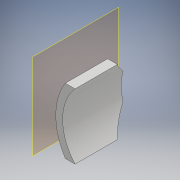
# Autodesk Inventor part: 15mm_radius_mold_with_crystal_skull
Saved by Autodesk Inventor 2018 (Build 220112000, 112)
## iProperties
Created: 2018-06-11
Part Number: 15mm_radius_mold_with_crystal_skull
Material: Generic
Document SubType Name: Modeling
Designer: McCormick Lab
Density: 1 g/cm^3
Appearance: Default
Author: McCormick Lab
Autodesk Inventor part; units mm, degrees
ref_plane "YZ Plane" through (0, 0, 0) normal (1, 0, 0) x (0, 1, 0)
ref_plane "XZ Plane" through (0, 0, 0) normal (0, 1, 0) x (-1, 0, 0)
ref_plane "XY Plane" through (0, 0, 0) normal (0, 0, 1) x (1, 0, 0)
sketch "Sketch1" plane through (0, 0, 0) normal (0, 1, 0) x (-1, 0, 0)
  arc A0 (0, -7.5) -> (0, 7.5) centre (0, 0) ccw
  line L0 (0, 7.5) -> (0, -7.5)
  dimension "d0" = 15
  constraints: 2 end point, 2 point on circle, 1 centre point, 1 coincident, 1 vertical
  measures "d0" diameter of A0
extrude "Extrusion1" add sketch "Sketch1" along normal blind 12
ref_plane "Work Plane1" through (-10, 0, 7.5) normal (1, 0, 0) x (0, 0, -1)
sketch "Sketch2" plane through (-10, 0, 7.5) normal (1, 0, 0) x (0, 0, -1)
  line L0 (2.5, 8.0057) -> (2.5, 1.5057)
  line L1 (2.5, 1.5057) -> (12.5, 1.5057)
  line L2 (12.5, 1.5057) -> (12.5, 8)
  line L3 (9.5, 10.5) -> (5.5, 10.5)
  line L4 (9.5, 10.5) -> (12.5, 8)
  line L5 (5.5, 10.5) -> (2.5, 8.0057)
  line L6 (15, 0) -> (15, 12) projected
  point P0 (7.5, 0)
  dimension "d9" = 10
  dimension "d10" = 6.5
  dimension "d12" = 4
  dimension "d14" = 3
  dimension "d15" = 3
  dimension "d24" = 2.5
  constraints: 12 end point, 1 horizontal, 1 parallel
  measures "d9" distance of L1.end L0.end
  measures "d10" distance of L0.end L0.start
  measures "d12" distance of L3.start L3.end
  measures "d14" horizontal distance of L0.end L3.end
  measures "d15" horizontal distance of L3.start L2.end
  measures "d24" distance between parallel lines of L6 L2
extrude "Extrusion2" add sketch "Sketch2" along normal blind 10
sketch "Sketch5" plane through (0, 0, 0) normal (0, 1, 0) x (-1, 0, 0)
  arc A0 (0, -7.5) -> (0, 7.5) centre (0, 0) ccw
  arc A1 (0, -7.5) -> (0, 7.5) centre (0, 0) ccw projected
  line L0 (0, 7.5) -> (0, -7.5)
  line L1 (0, -7.5) -> (0, 7.5)
  constraints: 4 end point, 2 point on circle, 1 centre point, 1 coincident
extrude "Extrusion5" cut sketch "Sketch5" along normal through all both and the other way through all
sketch "Sketch6" plane through (0, 0, 0) normal (0, 1, 0) x (-1, 0, 0)
  line L0 (7.0902, 5) -> (5.5902, 5)
  arc A0 (7.0902, -5) -> (7.0902, 5) centre (12.3734, 0) ccw
  arc A1 (7.0902, -5) -> (7.0902, 5) centre (-0.7358, 0) ccw
  point P0 (0, 0)
  constraints: 4 point on circle, 2 centre point, 2 end point, 1 horizontal
extrude "Extrusion6" cut sketch "Sketch6" along normal through all both and the other way through all
body "Solid1"
